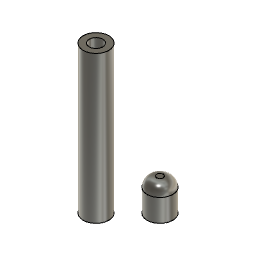
Skruer (Autodesk Fusion 360 design; units mm, degrees)
Autodesk Fusion 360 part; units mm, degrees
sketch "Sketch1" plane through (0, 0, 0) normal (0, 0, 1) x (1, 0, 0)
  circle A0 centre (10, 10) radius 4
  dimension "d2" = 8
  measures "d2" diameter of A0
extrude "Extrude1" add sketch "Sketch1" along normal blind 46 makes body 1
sketch "Sketch2" plane through (0, 0, 46) normal (0, 0, 1) x (-1, 0, 0)
  circle A0 centre (-10, -10) radius 4
  circle A1 centre (-10, -10) radius 2.1
  dimension "d5" = 4.2
  constraint concentric A0 A1
  measures "d5" diameter of A1
extrude "Extrude2" cut sketch "Sketch2" against normal blind 70 contours A1 bodies 1
sketch "Sketch3" plane through (0, 0, 0) normal (0, 0, 1) x (1, 0, 0)
  circle A0 centre (20, 20) radius 4
  dimension "d8" = 8
  measures "d8" diameter of A0
extrude "Extrude3" add sketch "Sketch3" along normal blind 10 separate body makes body 2
fillet "Fillet1" radius 3 1 edges at (16.2707, 18.5535, 10) on bodies 2
sketch "Sketch4" plane through (0, 0, 0) normal (0, 0, -1) x (1, 0, 0)
  circle A0 centre (20, -20) radius 4
  circle A1 centre (20, -20) radius 2.1
  dimension "d13" = 4.2
  constraint concentric A0 A1
  measures "d13" diameter of A1
extrude "Extrude4" cut sketch "Sketch4" against normal blind 5 contours A1 bodies 2
